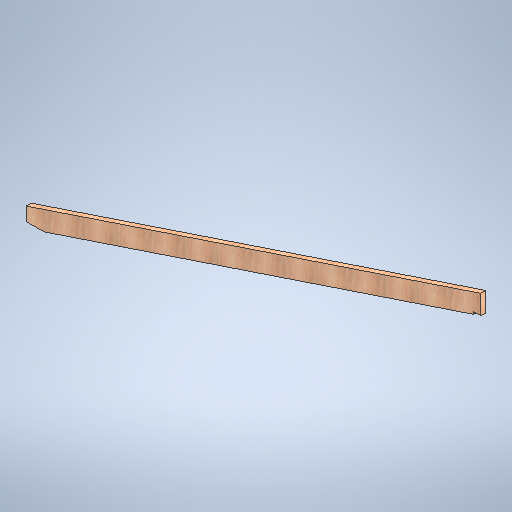
# Autodesk Inventor part: Rafter
Saved by Autodesk Inventor 2025.1 (Build 291241020, 241B)
## iProperties
Created: 2024-09-15
Part Number: Rafter
Material: Wood (Birch)
Document SubType Name: Modeling
Designer: Tom
Density: 0.55 g/cm^3
Appearance: Birch - Natural Polished
Author: Tom
Autodesk Inventor part; units mm, degrees
ref_plane "YZ Plane" through (0, 0, 0) normal (1, 0, 0) x (0, 1, 0)
ref_plane "XZ Plane" through (0, 0, 0) normal (0, 1, 0) x (-1, 0, 0)
ref_plane "XY Plane" through (0, 0, 0) normal (0, 0, 1) x (1, 0, 0)
sketch "Sketch1" plane through (0, 0, 0) normal (0, 0, 1) x (1, 0, 0)
  line L0 (0, 0) -> (3321.2278, 1108.1529)
  line L1 (3321.2278, 1255.4239) -> (-135.0962, 102.1952)
  line L2 (0, 0) -> (-135.0962, 0)
  line L3 (-135.0962, 0) -> (-135.0962, 102.1952)
  line L4 (-135.0962, 102.1952) -> (1593.1098, 678.8242)
  line L5 (3321.2278, 1108.1529) -> (3263.9, 1108.1529)
  line L6 (3321.2278, 1108.1529) -> (3321.2278, 1255.4239)
  line L7 (-88.9, 0) -> (-88.9, 117.6089)
  line L8 (3263.9, 1089.025) -> (3263.9, 1236.2961)
  line L9 (-135.0962, 102.1952) -> (-100.9981, 0)
  line L10 (-100.9981, 0) -> (25.6881, -379.689)
  dimension "d5" = 139.7
  dimension "d17" = 88.9
  dimension "d19" = 3352.8
  dimension "d23" = 57.3278
  dimension "d28" = 46.1962
  dimension "d33" = 1089.025
  dimension "d34" = 508
  dimension "d35" = 379.6891
  constraints: 22 end point, 6 point on line, 4 vertical, 2 coincident, 2 collinear, 2 horizontal, 1 perpendicular
  measures "d5" distance between parallel lines of L1 L0
  measures "d17" distance from line of L7 point (0, 0)
  measures "d19" distance between parallel lines of L7 L8
  measures "d23" distance between parallel lines of L6 L8
  measures "d28" distance between parallel lines of L3 L7
  measures "d33" vertical distance of L8.start point (0, 0)
  measures "d34" distance of L10.end L1.end
  measures "d35" vertical distance of L2.end L10.end
extrude "Extrusion1" add sketch "Sketch1" along normal blind 38.1 contours L2 L7 L1 L8 L0 | L2 L9 L1 L7 | L5 L8 L1 L6 | L2 L3 L9
ref_plane "Work Plane1" through (-135.0962, 102.1952, 0) normal (-0.948591, -0.3165046, 0) x (0.3165046, -0.948591, 0)
body "Solid1"
